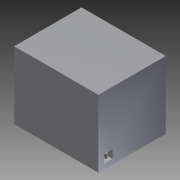
# Autodesk Inventor part: AC-DC converter
Saved by Autodesk Inventor 2012 (Build 160160000, 160)
## iProperties
Created: 2011-08-19
Part Number: AC-DC converter
Material: Default
Document SubType Name: Modeling
Designer: Minh Tran
Density: 1 g/cm^3
Author: Minh Tran
Autodesk Inventor part; units mm, degrees
ref_plane "YZ Plane" through (0, 0, 0) normal (1, 0, 0) x (0, 1, 0)
ref_plane "XZ Plane" through (0, 0, 0) normal (0, 1, 0) x (-1, 0, 0)
ref_plane "XY Plane" through (0, 0, 0) normal (0, 0, 1) x (1, 0, 0)
sketch "Sketch1" plane through (0, 0, 0) normal (0, 0, 1) x (1, 0, 0)
  line L0 (0, 0) -> (254, 0)
  line L1 (254, 0) -> (254, 203.2)
  line L2 (254, 203.2) -> (0, 203.2)
  line L3 (0, 203.2) -> (0, 0)
  dimension "d0" = 254
  dimension "d1" = 203.2
  constraints: 8 end point, 2 parallel, 1 horizontal, 1 perpendicular
  measures "d0" distance of L2.end L1.end
  measures "d1" distance of L1.end L0.end
extrude "Extrusion1" add sketch "Sketch1" along normal blind 203.2
sketch "Sketch3" plane through (254, 0, 0) normal (1, 0, 0) x (0, 0, -1)
  line L0 (-203.2, 203.2) -> (-203.2, 0) projected
  line L1 (0, 0) -> (-203.2, 0) projected
  line L2 (-185.9823, 14.7282) -> (-160.5823, 14.7282)
  line L3 (-160.5823, 14.7282) -> (-160.5823, 40.1282)
  line L4 (-160.5823, 40.1282) -> (-185.9823, 40.1282)
  line L5 (-185.9823, 40.1282) -> (-185.9823, 14.7282)
  dimension "d10" = 25.4
  dimension "d11" = 25.4
  dimension "d12" = 17.2177
  dimension "d13" = 14.7282
  constraints: 8 end point, 2 parallel, 1 horizontal, 1 perpendicular
  measures "d10" distance of L4.end L3.end
  measures "d11" distance of L3.end L2.end
  measures "d12" distance between parallel lines of L5 L0
  measures "d13" distance between parallel lines of L1 L2
extrude "Extrusion3" cut sketch "Sketch3" against normal blind 25.4
sketch "Sketch4" plane through (254, 14.7282, 185.9823) normal (0, 1, 0) x (1, 0, 0)
  circle A0 centre (-12.7, 4.7868) radius 3.81
  circle A1 centre (-12.7, 17.8785) radius 3.81
  point P0 (-254, 185.9823)
  dimension "d16" = 7.62
  dimension "d17" = 7.62
  constraints: 2 centre point
  measures "d16" diameter of A0
  measures "d17" diameter of A1
extrude "Extrusion4" add sketch "Sketch4" along normal blind 12.7
sketch "Sketch5" plane through (0, 0, 0) normal (-1, 0, 0) x (0, 0, 1)
  line L0 (0, 203.2) -> (0, 0) projected
  line L1 (0, 0) -> (203.2, 0) projected
  line L2 (16.7132, 14.732) -> (42.1132, 14.732)
  line L3 (42.1132, 14.732) -> (42.1132, 40.132)
  line L4 (42.1132, 40.132) -> (16.7132, 40.132)
  line L5 (16.7132, 40.132) -> (16.7132, 14.732)
  dimension "d20" = 25.4
  dimension "d21" = 25.4
  dimension "d22" = 16.7132
  dimension "d23" = 14.732
  constraints: 8 end point, 2 parallel, 1 horizontal, 1 perpendicular
  measures "d20" distance of L4.end L3.end
  measures "d21" distance of L3.end L2.end
  measures "d22" distance between parallel lines of L0 L5
  measures "d23" distance between parallel lines of L1 L2
extrude "Extrusion5" cut sketch "Sketch5" against normal blind 25.4
sketch "Sketch6" plane through (0, 14.732, 42.1132) normal (0, 1, 0) x (1, 0, 0)
  circle A0 centre (12.7, 20.3658) radius 3.81
  circle A1 centre (12.7, 6.9242) radius 3.81
  point P0 (0, 42.1132)
  dimension "d26" = 7.62
  dimension "d27" = 7.62
  constraints: 2 centre point
  measures "d26" diameter of A0
  measures "d27" diameter of A1
extrude "Extrusion6" add sketch "Sketch6" along normal blind 12.7
body "Solid1"
